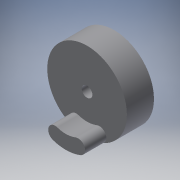
# Autodesk Inventor part: j024 output
Saved by Autodesk Inventor 2016 SP1 (Build 200210100, 210)
## iProperties
Created: 2016-09-17
Part Number: j024 output
Material: Generic
Document SubType Name: Modeling
Designer: benja
Density: 1 g/cm^3
Appearance: Default
Author: benja
Autodesk Inventor part; units mm, degrees
ref_plane "YZ Plane" through (0, 0, 0) normal (1, 0, 0) x (0, 1, 0)
ref_plane "XZ Plane" through (0, 0, 0) normal (0, 1, 0) x (-1, 0, 0)
ref_plane "XY Plane" through (0, 0, 0) normal (0, 0, 1) x (1, 0, 0)
sketch "Sketch1" plane through (0, 0, 0) normal (0, 0, 1) x (1, 0, 0)
  circle A0 centre (0, 0) radius 3.9 projected
  circle A1 centre (0, 0) radius 3.75
  dimension "d0" = 7.5
  constraints: 1 centre point, 1 coincident
  measures "d0" diameter of A1
extrude "Extrusion1" add sketch "Sketch1" along normal blind 2.55 contours A1
sketch "Sketch2" plane through (0, 0, 2.55) normal (0, 0, 1) x (1, 0, 0)
  arc A0 (-0.8017, -2.3151) -> (0.9206, -2.2705) centre (0, 0) ccw
  circle A1 centre (0, 0) radius 3.75 projected
  circle A2 centre (0, 0) radius 3.75 projected
  arc A3 (1.409, -3.4752) -> (0.9206, -2.2705) centre (1.1648, -2.8728) ccw
  arc A4 (-0.8017, -2.3151) -> (-1.2272, -3.5435) centre (-1.0145, -2.9293) ccw
  dimension "d3" = 1.3
  dimension "d4" = 3.48
  constraints: 10 point on circle, 4 tangent, 3 centre point, 1 concentric
  measures "d3" radial gap between concentric circles of A1 A0
extrude "Extrusion2" add sketch "Sketch2" along normal blind 2 contours A0 A3 A1 A4 picked at (-0.0123, -3.2943)
sketch "Sketch3" plane through (0, 0, 2.55) normal (0, 0, 1) x (1, 0, 0)
  circle A0 centre (0, 0) radius 0.5
  dimension "d7" = 1
  constraints: 1 centre point, 1 coincident
  measures "d7" diameter of A0
extrude "Extrusion3" cut sketch "Sketch3" against normal blind 2
body "Solid1"
